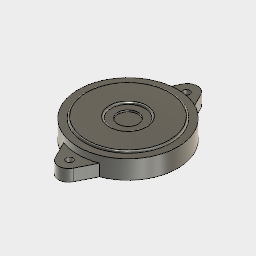
1739 Pizero Large (Autodesk Fusion 360 design; units mm, degrees)
Autodesk Fusion 360 part; units mm, degrees
note: some values were not read from the file. Set by a fixed rule: which sketch regions a step uses.
sketch "base" plane through (0, 0, 0) normal (0, 0, 1) x (1, 0, 0)
  circle A0 centre (0, 0) radius 14.65
  circle A1 centre (0, 17.2) radius 1
  line L0 (-5.25, 13.677) -> (-2.6683, 18.8354)
  arc A2 (2.6683, 18.8354) -> (-2.6683, 18.8354) centre (0, 17.5) ccw
  line L1 (2.6683, 18.8354) -> (5.25, 13.677)
  line L2 (0, 7.3551) -> (0, 15.8) construction
  line L3 (0, 0) -> (10, 0) construction
  dimension "d1" = 29.3
  dimension "d2" = 2
  dimension "d6" = 10.5
  dimension "d7" = 5.25
  dimension "d20" = 17.2
  measures "d1" diameter of A0
  measures "d2" diameter of A1
  measures "d6" distance of L0.start L1.end
  measures "d7" distance of L1.end L2
  measures "d20" distance of A1.centre L3
extrude "Extrude1" add sketch "base" along normal blind 6 contours A0
extrude "Extrude2" add sketch "base" along normal blind 3.5 contours A0 L0 A2 L1
sketch "top circles" plane through (0, 0, 6) normal (0, 0, 1) x (-1, 0, 0)
  circle A0 centre (0, 0) radius 14.65
  circle A1 centre (0, 0) radius 3
  circle A2 centre (0, 0) radius 5
  circle A3 centre (0, 0) radius 12.65
  dimension "d12" = 6
  dimension "d15" = 2
  dimension "d16" = 2
  measures "d12" diameter of A1
extrude "Extrude3" cut sketch "top circles" against normal blind 1 contours A1
extrude "Extrude4" cut sketch "top circles" against normal blind 0.5
fillet "Fillet1" radius 0.5 2 edges at (4.6616, -1.8081, 6) (11.7939, 4.5744, 6)
mirror "Mirror1" about plane through (0, 0, 0) normal (0, 1, 0) of "Extrude2"
equation "d7 = ( 10.5 / 2 ) * 1 mm"
equation "d20 = ( 34.4 / 2 ) * 1 mm"
